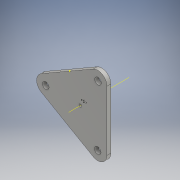
# Autodesk Inventor part: HandlePrimaryMirror
Saved by Autodesk Inventor 2019.4 (Build 234330000, 330)
## iProperties
Created: 2019-04-25
Part Number: HandlePrimaryMirror
Material: Aluminium 6061
Document SubType Name: Modeling
Designer: barto
Density: 2.7 g/cm^3
Appearance: Aluminium — płaski
Author: barto
Autodesk Inventor part; units mm, degrees
ref_plane "YZ Plane" through (0, 0, 0) normal (1, 0, 0) x (0, 1, 0)
ref_plane "XZ Plane" through (0, 0, 0) normal (0, 1, 0) x (-1, 0, 0)
ref_plane "XY Plane" through (0, 0, 0) normal (0, 0, 1) x (1, 0, 0)
sketch "Szkic1" plane through (0, 0, 0) normal (0, 1, 0) x (-1, 0, 0)
  line L0 (42.918, 0) -> (-17.7038, -35)
  line L1 (-17.7038, -35) -> (-17.7038, 35)
  line L2 (-17.7038, 35) -> (42.918, 0)
  point P0 (0, 0)
  dimension "d0" = 70
  dimension "d1" = 35
  dimension "d2" = 60
  dimension "d3" = 60
  constraints: 6 end point, 1 vertical
  measures "d0" distance of L0.end L1.end
  measures "d1" vertical distance of L1.end point (0, 0)
  measures "d2" angle of L1 L0
  measures "d3" angle of L1 L2
extrude "Wyciągnięcie proste1" add sketch "Szkic1" along normal blind 3
fillet "Zaokrąglenie1" radius 7 3 edges at (17.7038, 1.5, 35) (17.7038, 1.5, -35) (-42.918, 1.5, 0)
sketch "Szkic2" plane through (0, 3, 0) normal (0, 1, 0) x (1, 0, 0)
  circle A0 centre (10.92, -22.8756) radius 2.5
  arc A1 (7.2038, -28.9378) -> (17.7038, -22.8756) centre (10.7038, -22.8756) ccw projected
  circle A2 centre (-28.918, 0) radius 2.5
  circle A3 centre (10.7038, 23.0617) radius 2.5
  arc A4 (-32.418, 6.0622) -> (-32.418, -6.0622) centre (-28.918, 0) ccw projected
  arc A5 (17.7038, 22.8756) -> (7.2038, 28.9378) centre (10.7038, 22.8756) ccw projected
  point P0 (0, 0)
  dimension "d7" = 0
  dimension "d8" = 5
  dimension "d9" = 5
  dimension "d10" = 5
  dimension "d11" = 0
  dimension "d12" = 0
  constraints: 3 centre point
  measures "d7" vertical distance of A0.centre A1.centre
  measures "d8" diameter of A0
  measures "d9" diameter of A2
  measures "d10" diameter of A3
  measures "d11" distance of A2.centre A4.centre
  measures "d12" horizontal distance of A5.centre A3.centre
extrude "Wyciągnięcie proste2" cut sketch "Szkic2" against normal blind 3
sketch "Szkic3" plane through (0, 3, 0) normal (0, 1, 0) x (1, 0, 0)
  line L0 (7.2038, 28.9378) -> (-32.418, 6.0622) projected
  line L1 (-32.418, -6.0622) -> (7.2038, -28.9378) projected
  line L2 (7.2038, -28.9378) -> (-32.418, -6.0622) projected
  circle A0 centre (-2.5034, 0) radius 1
  point P0 (0, 0)
  point P1 (-12.6071, -17.5)
  point P2 (-12.6071, 17.5)
  dimension "d18" = 2
  constraints: 2 midpoint, 1 centre point
  measures "d18" diameter of A0
extrude "Wyciągnięcie proste3" cut sketch "Szkic3" against normal blind 3
sketch "Szkic4" plane through (-32.418, 0, 6.0622) normal (-0.5, 0, 0.8660254) x (0.8660254, 0, 0.5)
  point P0 (25.0437, 0)
sketch "Szkic5" plane through (0, 3, 0) normal (0, 1, 0) x (1, 0, 0)
  circle A0 centre (-2.5034, 0) radius 1 projected
  line L0 (-3.5034, 0) -> (-3.5034, -1.2647)
  point P0 (0, 0)
  dimension "d19" = 1
  constraints: 2 end point, 1 vertical
  measures "d19" distance of A0.centre L0.start
ref_plane "Płaszczyzna konstrukcyjna1" through (-3.5034, 3, 0) normal (0, 0, 1) x (1, 0, 0)
sketch "Szkic6" plane through (0, 3, 0) normal (0, 1, 0) x (1, 0, 0)
  point P0 (0, 0)
sketch "Szkic7" plane through (-3.5034, 3, 0) normal (0, 0, 1) x (1, 0, 0)
  line L0 (0, 0) -> (2, 0) projected
  line L1 (1, 0) -> (-1.5981, 0)
  line L2 (1, -1.5) -> (-1.5981, 0)
  line L3 (1, -1.5) -> (1, 0)
  line L4 (1, 0.6) -> (1, -3.6) projected
  point P0 (3.5034, -3)
  dimension "d20" = 1.5
  dimension "d21" = 60
  constraints: 6 end point, 1 horizontal, 1 midpoint, 1 vertical
  measures "d20" distance of L1.start L2.start
  measures "d21" angle of L3 L2
revolve "Obrót1" cut sketch "Szkic7" angle 360 about axis through (-2.5034, 3, 0) along (0, -1, 0)
sketch "Szkic8" plane through (0, 3, 0) normal (0, 1, 0) x (1, 0, 0)
  point P0 (0, 0)
